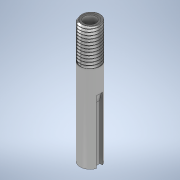
# Autodesk Inventor part: Tornillo deslizante
Saved by Autodesk Inventor 2020 (Build 240168000, 168)
## iProperties
Created: 2020-09-17
Part Number: Tornillo deslizante
Material: Steel AISI 1045 HV HR
Document SubType Name: Modeling
Designer: aaron
Density: 7.85 g/cm^3
Appearance: Steel Doors - Painted White
Author: aaron
Autodesk Inventor part; units mm, degrees
ref_plane "YZ Plane" through (0, 0, 0) normal (1, 0, 0) x (0, 1, 0)
ref_plane "XZ Plane" through (0, 0, 0) normal (0, 1, 0) x (-1, 0, 0)
ref_plane "XY Plane" through (0, 0, 0) normal (0, 0, 1) x (1, 0, 0)
sketch "Sketch1" plane through (0, 0, 0) normal (0, 1, 0) x (-1, 0, 0)
  circle A0 centre (0, 0) radius 7.9248
  dimension "d0" = 15.8496
  constraints: 1 centre point, 1 coincident
  measures "d0" diameter of A0
extrude "Extrusion1" add sketch "Sketch1" along normal blind 98.425
sketch "Sketch2" plane through (0, 98.425, 0) normal (0, 1, 0) x (1, 0, 0)
  circle A0 centre (0, 0) radius 4.7498
  dimension "d3" = 9.4996
  constraints: 1 centre point, 1 coincident
  measures "d3" diameter of A0
extrude "Extrusion2" cut sketch "Sketch2" against normal blind 50.8
thread "Thread1" size "5/8-11 UNC" class "2A" standard "ANSI Unified Screw Threads" length 28.575
sketch "Sketch3" plane through (0, 0, 0) normal (0, -1, 0) x (1, 0, 0)
  line L0 (-11.0947, 0) -> (11.0947, 0) projected
  circle A0 centre (0, 0) radius 7.9248 projected
  line L1 (7.9248, 0) -> (5.5435, 0) construction
  line L2 (5.5435, 0) -> (5.5435, -2.3813)
  line L3 (5.5435, -2.3813) -> (7.5586, -2.3813)
  line L4 (5.5435, 0) -> (5.5435, 2.3813)
  line L5 (5.5435, 2.3813) -> (7.5586, 2.3813)
  dimension "d8" = 2.3813
  dimension "d9" = 2.3813
  constraints: 10 end point, 2 point on circle, 2 point on line, 2 symmetric about line, 1 horizontal, 1 vertical
  measures "d8" distance of L1.end L1.start
  measures "d9" distance between parallel lines of L0 L3
extrude "Extrusion3" cut sketch "Sketch3" against normal blind 50.8 contours L4 L5 A0 L0 | L0 A0 L3 L2 picked at (6.2828, 1.3275) picked at (6.2828, -1.3275)
fillet "Fillet1" radius 11.1125 1 edges at (5.5435, 50.8, 0)
sketch "Sketch5" plane through (0, 98.425, 0) normal (1, 0, 0) x (0, 0, 1)
  line L0 (7.9248, 0) -> (7.9248, 28.575)
  line L1 (7.9248, 28.575) -> (6.2127, 28.575)
  line L2 (6.2127, 28.575) -> (6.2127, 0)
  line L3 (6.2127, 0) -> (7.9248, 0)
  line L4 (0, -22.7065) -> (0, 118.6136) projected
  constraints: 8 end point
revolve "Revolution1" cut sketch "Sketch5" angle 360 about axis through (0, 98.425, 0) along (0, -1, 0)
sketch "Sketch6" plane through (0, 98.425, 0) normal (1, 0, 0) x (0, 0, 1)
  line L0 (7.9248, 0) -> (7.9248, 28.575)
  line L1 (7.9248, 28.575) -> (6.2127, 28.575)
  line L2 (6.2127, 28.575) -> (6.2127, 0)
  line L3 (6.2127, 0) -> (7.9248, 0)
  line L4 (0, -22.7065) -> (0, 118.6136) projected
  constraints: 8 end point
revolve "Revolution2" add sketch "Sketch6" angle 360 about axis through (0, 98.425, 0) along (0, -1, 0) separate body
sketch "Sketch4" plane through (0, 98.425, 0) normal (-1, 0, 0) x (0, -1, 0)
  line L0 (-1.3471, -6.3296) -> (-1.1546, -6.3296) construction
  line L1 (0.1923, -7.8082) -> (-0.0001, -8.1778) construction
  line L2 (-2.3092, -8.1778) -> (-2.5016, -7.8082) construction
  line L3 (-0.9622, -6.3296) -> (-1.1546, -5.96) construction
  line L4 (-1.1546, -5.96) -> (-1.3471, -6.3296) construction
  line L5 (-2.3092, -8.1778) -> (-2.1168, -7.8082) construction
  line L6 (-0.9622, -6.3296) -> (-0.1925, -7.8082)
  line L7 (-2.5016, -7.8082) -> (-2.1168, -7.8082) construction
  arc A0 (-2.5016, -7.8082) -> (-2.3092, -7.925) centre (-2.3092, -7.708) ccw construction
  line L8 (0.1923, -7.8082) -> (-0.1925, -7.8082) construction
  line L9 (-2.3092, -8.1778) -> (-2.3092, -7.8082) construction
  line L10 (-0.0001, -8.1778) -> (-0.0001, -7.8082) construction
  line L11 (-1.1546, -5.96) -> (-1.1546, -6.2129) construction
  line L12 (-2.3092, -7.925) -> (-0.0001, -7.925)
  arc A1 (-2.3092, -7.925) -> (-2.1168, -7.8082) centre (-2.3092, -7.708) ccw
  line L13 (-0.1925, -7.8082) -> (-0.0001, -8.1778) construction
  line L14 (-2.1168, -7.8082) -> (-1.3471, -6.3296)
  line L15 (-0.0001, -0.0002) -> (-0.0001, 0.0177)
  line L16 (-0.0001, 0.0177) -> (-0.0001, -0.0002)
  line L17 (-0.0001, -0.0002) -> (0.0334, -0.0002)
  arc A2 (-0.1925, -7.8082) -> (-0.0001, -7.925) centre (-0.0001, -7.708) ccw
  arc A3 (-0.0001, -7.925) -> (0.1923, -7.8082) centre (-0.0001, -7.708) ccw construction
  arc A4 (-1.1546, -6.2129) -> (-1.3471, -6.3296) centre (-1.1546, -6.4298) ccw
  arc A5 (-0.9622, -6.3296) -> (-1.1546, -6.2129) centre (-1.1546, -6.4298) ccw
  line L18 (-1.1546, -6.2129) -> (-1.1546, -6.3296) construction
  line L19 (-1.1546, -6.3296) -> (-0.9622, -6.3296) construction
  dimension "d13" = 55
  dimension "d14" = 0.3696
  dimension "d15" = 0.3696
  dimension "Sketch4_ThreadOffset" = 0
  dimension "Sketch4_MajorRadius" = 7.9248
  dimension "d18" = 2.3091
  dimension "Sketch4_MinorRadius" = 6.2127
  constraints: 40 end point, 12 point on circle, 10 parallel, 8 tangent, 6 centre point, 6 collinear, 2 midpoint, 2 point on line, 1 horizontal, 1 perpendicular, 3 other
  measures "d13" angle of L6 L14
  measures "d14" distance of L3.end L0.end
  measures "d15" distance of L1.end L10.end
  measures "Sketch4_ThreadOffset" distance between parallel lines of L15 L10
  measures "Sketch4_MajorRadius" distance from line of L12 L15.start
  measures "d18" distance from line of L1.end L9
  measures "Sketch4_MinorRadius" distance edge to line of A5 L17
coil "Coil1" sketch "Sketch4" operation cut axis through (0, 98.425, 0) along (0, -1, 0) pitch 2.3114 turns 14.360639 hand right bodies 2
equation "\"d13\" = d20"
equation "\"d14\" = 0.160083 * Sketch4_Pitch"
equation "\"d15\" = 0.160083 * Sketch4_Pitch"
equation "\"d18\" = Sketch4_Pitch"
equation "\"d20\" = 55deg"
equation "\"Sketch4_Pitch\" = 2.30909"
body "Solid1"
body "Solid2"
